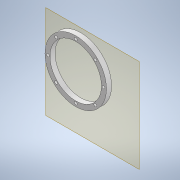
# Autodesk Inventor part: upper_plate
Saved by Autodesk Inventor 2022 (Build 260153000, 153)
## iProperties
Created: 2022-03-16
Part Number: upper_plate
Material: Generic
Document SubType Name: Modeling
Designer: zac-h
Density: 1 g/cm^3
Appearance: Default
Author: zac-h
Autodesk Inventor part; units mm, degrees
ref_plane "YZ Plane" through (0, 0, 0) normal (1, 0, 0) x (0, 1, 0)
ref_plane "XZ Plane" through (0, 0, 0) normal (0, 1, 0) x (-1, 0, 0)
ref_plane "XY Plane" through (0, 0, 0) normal (0, 0, 1) x (1, 0, 0)
ref_plane "Work Plane1" through (0, 0, 0) normal (0, 0, 1) x (1, 0, 0)
sketch "Sketch1" plane through (0, 0, 0) normal (0, 0, 1) x (1, 0, 0)
  circle A0 centre (11.7233, 46.6483) radius 2.132 projected
  circle A1 centre (20.0025, 56.1975) radius 2.132 projected
  circle A2 centre (32.7025, 56.1975) radius 2.132 projected
  circle A3 centre (45.4025, 56.1975) radius 2.132 projected
  circle A4 centre (58.1025, 56.1975) radius 2.132 projected
  circle A5 centre (-58.7375, 17.4625) radius 2.132 projected
  circle A6 centre (-46.6483, 46.6483) radius 2.132 projected
  circle A7 centre (-17.4625, 58.7375) radius 2.132 projected
  circle A8 centre (11.7233, 46.6483) radius 2.132 projected
  circle A9 centre (23.8125, 17.4625) radius 2.132 projected
  circle A10 centre (11.7233, -11.7233) radius 2.132 projected
  circle A11 centre (-17.4625, -23.8125) radius 2.132 projected
  circle A12 centre (-46.6483, -11.7233) radius 2.132 projected
  circle A13 centre (-56.1975, -32.7025) radius 2.132 projected
  circle A14 centre (-56.1975, -45.4025) radius 2.132 projected
  circle A15 centre (-56.1975, -58.1025) radius 2.132 projected
  circle A16 centre (-56.1975, -20.0025) radius 2.132 projected
  circle A17 centre (-17.4625, 17.4625) radius 38.1 projected
  circle A18 centre (-17.4625, 17.4625) radius 38.3
  circle A19 centre (-17.4625, 17.4625) radius 45.72
  circle A20 centre (-17.4625, 17.4625) radius 32.55 projected
  line L0 (9.485, -18.7266) -> (-48.7269, -62.0728) projected
  arc A21 (9.485, -18.7266) -> (18.7266, -9.485) centre (-17.4625, 17.4625) ccw projected
  line L1 (62.0728, 48.7269) -> (18.7266, -9.485) projected
  arc A22 (62.0728, 48.7269) -> (62.5825, 50.2648) centre (60.0075, 50.2648) ccw projected
  line L2 (62.5825, 60.0075) -> (62.5825, 50.2648) projected
  arc A23 (62.5825, 60.0075) -> (60.0075, 62.5825) centre (60.0075, 60.0075) ccw projected
  line L3 (-17.4625, 62.5825) -> (60.0075, 62.5825) projected
  arc A24 (-17.4625, 62.5825) -> (-62.5825, 17.4625) centre (-17.4625, 17.4625) ccw projected
  line L4 (-62.5825, -60.0075) -> (-62.5825, 17.4625) projected
  arc A25 (-62.5825, -60.0075) -> (-60.0075, -62.5825) centre (-60.0075, -60.0075) ccw projected
  line L5 (-50.2648, -62.5825) -> (-60.0075, -62.5825) projected
  arc A26 (-50.2648, -62.5825) -> (-48.7269, -62.0728) centre (-50.2648, -60.0075) ccw projected
  arc A27 (-46.4955, -21.6632) -> (-38.635, -17.6063) centre (-46.6483, -11.7233) ccw projected
  arc A28 (-33.9418, -16.445) -> (-38.635, -17.6063) centre (-35.592, -19.8403) ccw projected
  arc A29 (-33.9418, -16.445) -> (-29.7861, -18.1664) centre (-17.4625, 17.4625) ccw projected
  arc A30 (-27.2887, -22.3061) -> (-29.7861, -18.1664) centre (-31.0201, -21.734) ccw projected
  arc A31 (-27.2887, -22.3061) -> (-26.8535, -27.0731) centre (-17.4625, -23.8125) ccw projected
  arc A32 (-28.1651, -31.3391) -> (-26.8535, -27.0731) centre (-30.4197, -28.3113) ccw projected
  line L6 (-44.1828, -43.2664) -> (-28.1651, -31.3391) projected
  arc A33 (-50.2124, -40.2386) -> (-44.1828, -43.2664) centre (-46.4374, -40.2386) ccw projected
  line L7 (-50.2124, -25.4377) -> (-50.2124, -40.2386) projected
  arc A34 (-46.4955, -21.6632) -> (-50.2124, -25.4377) centre (-46.4374, -25.4377) ccw projected
  line L8 (40.2386, 50.2124) -> (25.4377, 50.2124) projected
  arc A35 (43.2664, 44.1828) -> (40.2386, 50.2124) centre (40.2386, 46.4374) ccw projected
  line L9 (31.3391, 28.1651) -> (43.2664, 44.1828) projected
  arc A36 (27.0731, 26.8535) -> (31.3391, 28.1651) centre (28.3113, 30.4197) ccw projected
  arc A37 (27.0731, 26.8535) -> (22.3061, 27.2887) centre (23.8125, 17.4625) ccw projected
  arc A38 (18.1664, 29.7861) -> (22.3061, 27.2887) centre (21.734, 31.0201) ccw projected
  arc A39 (18.1664, 29.7861) -> (16.445, 33.9418) centre (-17.4625, 17.4625) ccw projected
  arc A40 (17.6063, 38.635) -> (16.445, 33.9418) centre (19.8403, 35.592) ccw projected
  arc A41 (17.6063, 38.635) -> (21.6632, 46.4955) centre (11.7233, 46.6483) ccw projected
  arc A42 (25.4377, 50.2124) -> (21.6632, 46.4955) centre (25.4377, 46.4374) ccw projected
  point P0 (0, 0)
  dimension "d0" = 0.2
  constraints: 2 centre point, 1 coincident
  measures "d0" radial gap between concentric circles of A17 A18
extrude "Extrusion1" add sketch "Sketch1" along normal blind 7.6 contours A38 A37 A36 A19 L1 A21 L0 A32 A31 A30 A18 | A18 A40 A41 A19 A36 A37 A38 | A30 A31 A32 A19 A27 A28 A18 | A18 A28 A27 A19 L4 A24 L3 A41 A40 | L3 A24 L4 A19 | L0 A21 L1 A19
body "Solid1"
